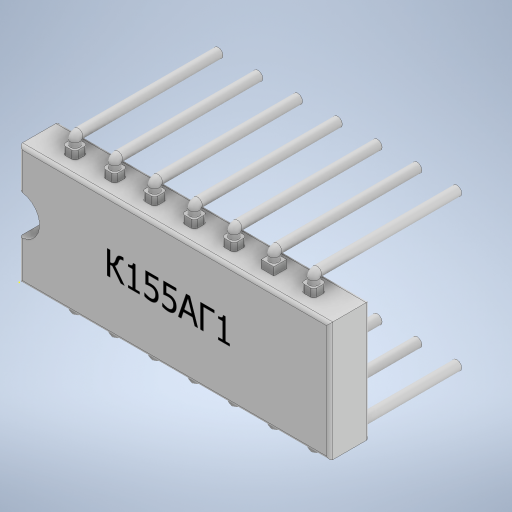
# Autodesk Inventor part: К155АГ1
Saved by Autodesk Inventor 2024 (Build 280153000, 153)
## iProperties
Created: 2023-12-19
Part Number: К155АГ1
Material: Generic
Document SubType Name: Sheet Metal
Designer: user
Density: 1 g/cm^3
Sheet Metal Rule: Default
Appearance: Default
Author: user
Autodesk Inventor part; units mm, degrees
sketch "Sketch1" plane through (0, 0, 0) normal (0, 0, 1) x (1, 0, 0)
  line L0 (0, 0) -> (495.3, 0)
  line L1 (495.3, 0) -> (495.3, 190.5)
  line L2 (495.3, 190.5) -> (0, 190.5)
  line L3 (0, 190.5) -> (0, 127)
  line L4 (0, 0) -> (0, 63.5)
  arc A0 (0, 63.5) -> (0, 127) centre (0.6755, 95.25) ccw
  line L5 (0, 190.5) -> (57.15, 190.5)
  line L6 (57.15, 190.5) -> (57.15, 203.2)
  line L7 (46.99, 203.2) -> (67.31, 203.2)
  line L8 (67.31, 203.2) -> (67.31, 190.5)
  line L9 (67.31, 190.5) -> (46.99, 190.5)
  line L10 (46.99, 190.5) -> (46.99, 203.2)
  line L11 (57.15, 203.2) -> (120.65, 203.2)
  line L12 (120.65, 203.2) -> (184.15, 203.2)
  line L13 (184.15, 203.2) -> (247.65, 203.2)
  line L14 (247.65, 203.2) -> (311.15, 203.2)
  line L15 (311.15, 203.2) -> (374.65, 203.2)
  line L16 (374.65, 203.2) -> (438.15, 203.2)
  line L17 (438.15, 203.2) -> (495.3, 203.2)
  line L18 (120.65, 203.2) -> (110.49, 203.2)
  line L19 (110.49, 203.2) -> (110.49, 190.5)
  line L20 (110.49, 190.5) -> (120.65, 190.5)
  line L21 (120.65, 190.5) -> (120.65, 203.2)
  line L22 (120.65, 203.2) -> (130.81, 203.2)
  line L23 (130.81, 203.2) -> (130.81, 190.5)
  line L24 (130.81, 190.5) -> (120.65, 190.5)
  line L25 (120.65, 190.5) -> (120.65, 203.2)
  line L26 (184.15, 203.2) -> (173.99, 203.2)
  line L27 (173.99, 203.2) -> (173.99, 190.5)
  line L28 (173.99, 190.5) -> (184.15, 190.5)
  line L29 (184.15, 190.5) -> (184.15, 203.2)
  line L30 (184.15, 203.2) -> (194.31, 203.2)
  line L31 (194.31, 203.2) -> (194.31, 190.5)
  line L32 (194.31, 190.5) -> (184.15, 190.5)
  line L33 (184.15, 190.5) -> (184.15, 203.2)
  line L34 (247.65, 203.2) -> (237.49, 203.2)
  line L35 (237.49, 203.2) -> (237.49, 190.5)
  line L36 (237.49, 190.5) -> (247.65, 190.5)
  line L37 (247.65, 190.5) -> (247.65, 203.2)
  line L38 (247.65, 203.2) -> (257.81, 203.2)
  line L39 (257.81, 203.2) -> (257.81, 190.5)
  line L40 (257.81, 190.5) -> (247.65, 190.5)
  line L41 (247.65, 190.5) -> (247.65, 203.2)
  line L42 (311.15, 203.2) -> (300.99, 203.2)
  line L43 (300.99, 203.2) -> (300.99, 190.5)
  line L44 (300.99, 190.5) -> (311.15, 190.5)
  line L45 (311.15, 190.5) -> (311.15, 203.2)
  line L46 (311.15, 203.2) -> (321.31, 203.2)
  line L47 (321.31, 203.2) -> (321.31, 190.5)
  line L48 (321.31, 190.5) -> (311.15, 190.5)
  line L49 (311.15, 190.5) -> (311.15, 203.2)
  line L50 (374.65, 203.2) -> (384.81, 203.2)
  line L51 (384.81, 203.2) -> (384.81, 190.5)
  line L52 (384.81, 190.5) -> (374.65, 190.5)
  line L53 (374.65, 190.5) -> (374.65, 203.2)
  line L54 (374.65, 203.2) -> (364.49, 203.2)
  line L55 (364.49, 203.2) -> (364.49, 190.5)
  line L56 (364.49, 190.5) -> (374.65, 190.5)
  line L57 (374.65, 190.5) -> (374.65, 203.2)
  line L58 (438.15, 203.2) -> (448.31, 203.2)
  line L59 (448.31, 203.2) -> (448.31, 190.5)
  line L60 (448.31, 190.5) -> (438.15, 190.5)
  line L61 (438.15, 190.5) -> (438.15, 203.2)
  line L62 (438.15, 203.2) -> (427.99, 203.2)
  line L63 (427.99, 203.2) -> (427.99, 190.5)
  line L64 (427.99, 190.5) -> (438.15, 190.5)
  line L65 (438.15, 190.5) -> (438.15, 203.2)
  line L66 (0, 0) -> (57.15, 0)
  line L67 (57.15, 0) -> (120.65, 0)
  line L68 (120.65, 0) -> (184.15, 0)
  line L69 (184.15, 0) -> (247.65, 0)
  line L70 (247.65, 0) -> (311.15, 0)
  line L71 (311.15, 0) -> (374.65, 0)
  line L72 (374.65, 0) -> (438.15, 0)
  line L73 (438.15, 0) -> (495.3, 0)
  line L74 (57.15, 0) -> (46.99, 0)
  line L75 (46.99, 0) -> (46.99, -12.7)
  line L76 (46.99, -12.7) -> (57.15, -12.7)
  line L77 (57.15, -12.7) -> (57.15, 0)
  line L78 (57.15, 0) -> (67.31, 0)
  line L79 (67.31, 0) -> (67.31, -12.7)
  line L80 (67.31, -12.7) -> (57.15, -12.7)
  line L81 (57.15, -12.7) -> (57.15, 0)
  line L82 (120.65, 0) -> (110.49, 0)
  line L83 (110.49, 0) -> (110.49, -12.7)
  line L84 (110.49, -12.7) -> (120.65, -12.7)
  line L85 (120.65, -12.7) -> (120.65, 0)
  line L86 (120.65, 0) -> (130.81, 0)
  line L87 (130.81, 0) -> (130.81, -12.7)
  line L88 (130.81, -12.7) -> (120.65, -12.7)
  line L89 (120.65, -12.7) -> (120.65, 0)
  line L90 (184.15, 0) -> (194.31, 0)
  line L91 (194.31, 0) -> (194.31, -12.7)
  line L92 (194.31, -12.7) -> (184.15, -12.7)
  line L93 (184.15, -12.7) -> (184.15, 0)
  line L94 (184.15, 0) -> (173.99, 0)
  line L95 (173.99, 0) -> (173.99, -12.7)
  line L96 (173.99, -12.7) -> (184.15, -12.7)
  line L97 (184.15, -12.7) -> (184.15, 0)
  line L98 (247.65, 0) -> (257.81, 0)
  line L99 (257.81, 0) -> (257.81, -12.7)
  line L100 (257.81, -12.7) -> (247.65, -12.7)
  line L101 (247.65, -12.7) -> (247.65, 0)
  line L102 (247.65, 0) -> (237.49, 0)
  line L103 (237.49, 0) -> (237.49, -12.7)
  line L104 (237.49, -12.7) -> (247.65, -12.7)
  line L105 (247.65, -12.7) -> (247.65, 0)
  line L106 (311.15, 0) -> (321.31, 0)
  line L107 (321.31, 0) -> (321.31, -12.7)
  line L108 (321.31, -12.7) -> (311.15, -12.7)
  line L109 (311.15, -12.7) -> (311.15, 0)
  line L110 (311.15, 0) -> (300.99, 0)
  line L111 (300.99, 0) -> (300.99, -12.7)
  line L112 (300.99, -12.7) -> (311.15, -12.7)
  line L113 (311.15, -12.7) -> (311.15, 0)
  line L114 (374.65, 0) -> (384.81, 0)
  line L115 (384.81, 0) -> (384.81, -12.7)
  line L116 (384.81, -12.7) -> (374.65, -12.7)
  line L117 (374.65, -12.7) -> (374.65, 0)
  line L118 (374.65, 0) -> (364.49, 0)
  line L119 (364.49, 0) -> (364.49, -12.7)
  line L120 (364.49, -12.7) -> (374.65, -12.7)
  line L121 (374.65, -12.7) -> (374.65, 0)
  line L122 (438.15, 0) -> (448.31, 0)
  line L123 (448.31, 0) -> (448.31, -12.7)
  line L124 (448.31, -12.7) -> (438.15, -12.7)
  line L125 (438.15, -12.7) -> (438.15, 0)
  line L126 (438.15, 0) -> (427.99, 0)
  line L127 (427.99, 0) -> (427.99, -12.7)
  line L128 (427.99, -12.7) -> (438.15, -12.7)
  line L129 (438.15, -12.7) -> (438.15, 0)
  dimension "d0" = 495.3
  dimension "d1" = 190.5
  dimension "d2" = 495.3
  dimension "d3" = 63.5
  dimension "d4" = 63.5
  dimension "d5" = 57.15
  dimension "d6" = 12.7
  dimension "d8" = 10.16
  dimension "d9" = 63.5
  dimension "d10" = 63.5
  dimension "d11" = 63.5
  dimension "d12" = 63.5
  dimension "d13" = 63.5
  dimension "d14" = 63.5
  dimension "d15" = 57.15
  dimension "d16" = 10.16
  dimension "d17" = 12.7
  dimension "d18" = 10.16
  dimension "d19" = 12.7
  dimension "d20" = 10.16
  dimension "d21" = 10.16
  dimension "d22" = 12.7
  dimension "d23" = 10.16
  dimension "d24" = 12.7
  dimension "d25" = 10.16
  dimension "d26" = 12.7
  dimension "d27" = 10.16
  dimension "d28" = 12.7
  dimension "d29" = 10.16
  dimension "d30" = 12.7
  dimension "d31" = 10.16
  dimension "d32" = 12.7
  dimension "d33" = 10.16
  dimension "d34" = 12.7
  dimension "d35" = 10.16
  dimension "d36" = 12.7
  dimension "d37" = 10.16
  dimension "d38" = 12.7
  dimension "d39" = 57.15
  dimension "d40" = 63.5
  dimension "d41" = 63.5
  dimension "d42" = 63.5
  dimension "d43" = 63.5
  dimension "d44" = 63.5
  dimension "d45" = 63.5
  dimension "d46" = 57.15
  dimension "d47" = 10.16
  dimension "d48" = 12.7
  dimension "d49" = 10.16
  dimension "d50" = 12.7
  dimension "d51" = 10.16
  dimension "d52" = 12.7
  dimension "d53" = 10.16
  dimension "d54" = 12.7
  dimension "d55" = 10.16
  dimension "d56" = 12.7
  dimension "d57" = 10.16
  dimension "d58" = 12.7
  dimension "d59" = 10.16
  dimension "d60" = 12.7
  dimension "d61" = 10.16
  dimension "d62" = 12.7
  dimension "d63" = 10.16
  dimension "d64" = 12.7
  constraints: 258 end point, 54 parallel, 30 perpendicular, 27 horizontal, 9 point on line, 3 vertical, 2 point on circle, 1 centre point, 1 collinear, 10 other
  measures "d0" distance of L4.start L1.start
  measures "d1" distance of L1.start L1.end
  measures "d2" distance of L1.end L2.end
  measures "d3" distance of L2.end L3.end
  measures "d4" distance of L4.start L4.end
  measures "d5" distance of L2.end L5.end
  measures "d6" distance of L5.end L6.end
  measures "d8" distance of L6.end L7.start
  measures "d9" distance of L6.end L11.end
  measures "d10" distance of L11.end L12.end
  measures "d11" distance of L12.end L13.end
  measures "d12" distance of L13.end L14.end
  measures "d13" distance of L14.end L15.end
  measures "d14" distance of L15.end L16.end
  measures "d15" distance of L16.end L17.end
  measures "d16" distance of L20.end L19.end
  measures "d17" distance of L19.end L18.end
  measures "d18" distance of L23.end L24.end
  measures "d19" distance of L22.end L23.end
  measures "d20" distance of L28.end L27.end
  measures "d21" distance of L31.end L32.end
  measures "d22" distance of L30.end L31.end
  measures "d23" distance of L36.end L35.end
  measures "d24" distance of L35.end L34.end
  measures "d25" distance of L39.end L40.end
  measures "d26" distance of L38.end L39.end
  measures "d27" distance of L44.end L43.end
  measures "d28" distance of L43.end L42.end
  measures "d29" distance of L47.end L48.end
  measures "d30" distance of L46.end L47.end
  measures "d31" distance of L51.end L52.end
  measures "d32" distance of L50.end L51.end
  measures "d33" distance of L56.end L55.end
  measures "d34" distance of L55.end L54.end
  measures "d35" distance of L59.end L60.end
  measures "d36" distance of L58.end L59.end
  measures "d37" distance of L64.end L63.end
  measures "d38" distance of L63.end L62.end
  measures "d39" distance of L4.start L66.end
  measures "d40" distance of L66.end L67.end
  measures "d41" distance of L67.end L68.end
  measures "d42" distance of L68.end L69.end
  measures "d43" distance of L69.end L70.end
  measures "d44" distance of L70.end L71.end
  measures "d45" distance of L71.end L72.end
  measures "d46" distance of L72.end L1.start
  measures "d47" distance of L76.end L75.end
  measures "d48" distance of L75.end L74.end
  measures "d49" distance of L79.end L80.end
  measures "d50" distance of L78.end L79.end
  measures "d51" distance of L84.end L83.end
  measures "d52" distance of L83.end L82.end
  measures "d53" distance of L87.end L88.end
  measures "d54" distance of L86.end L87.end
  measures "d55" distance of L91.end L92.end
  measures "d56" distance of L90.end L91.end
  measures "d57" distance of L96.end L95.end
  measures "d58" distance of L95.end L94.end
  measures "d59" distance of L99.end L100.end
  measures "d60" distance of L98.end L99.end
  measures "d61" distance of L104.end L103.end
  measures "d62" distance of L103.end L102.end
  measures "d63" distance of L107.end L108.end
  measures "d64" distance of L106.end L107.end
extrude "Extrusion1" add sketch "Sketch1" along normal mid plane 63.5 contours L4 A0 L3 L2 L1 L0
extrude "Extrusion2" add sketch "Sketch1" along normal mid plane 20.32 contours L0 L77 L76 L75 | L0 L79 L80 L77 | L0 L85 L84 L83 | L10 L7 L6 L2 | L0 L87 L88 L85 | L6 L7 L8 L2 | L0 L93 L96 L95 | L19 L11 L21 L2 | L0 L91 L92 L93 | L21 L12 L23 L2 | L0 L101 L104 L103 | L27 L12 L29 L2 | L0 L99 L100 L101 | L29 L13 L31 L2 | L0 L109 L112 L111 | L35 L13 L37 L2 | L0 L107 L108 L109 | L37 L14 L39 L2 | L0 L117 L120 L119 | L43 L14 L45 L2 | L0 L115 L116 L117 | L45 L15 L47 L2 | L0 L125 L128 L127 | L55 L15 L53 L2 | L0 L123 L124 L125 | L53 L16 L51 L2 | L63 L16 L61 L2 | L61 L17 L59 L2
fillet "Fillet1" radius 5.08 62 edges at (67.31, 196.85, 10.16) (67.31, 196.85, -10.16) (46.99, 196.85, -10.16) (46.99, 196.85, 10.16) (110.49, 196.85, 10.16) (130.81, 196.85, 10.16) (110.49, 196.85, -10.16) (130.81, 196.85, -10.16) (173.99, 196.85, 10.16) (173.99, 196.85, -10.16) (194.31, 196.85, -10.16) (194.31, 196.85, 10.16) (237.49, 196.85, 10.16) (257.81, 196.85, 10.16) (237.49, 196.85, -10.16) (257.81, 196.85, -10.16) (300.99, 196.85, 10.16) (321.31, 196.85, 10.16) (300.99, 196.85, -10.16) (321.31, 196.85, -10.16) (427.99, 196.85, 10.16) (448.31, 196.85, 10.16) (448.31, 196.85, -10.16) (427.99, 196.85, -10.16) (46.99, -6.35, 10.16) (46.99, -6.35, -10.16) (67.31, -6.35, -10.16) (67.31, -6.35, 10.16) (110.49, -6.35, 10.16) (110.49, -6.35, -10.16) (130.81, -6.35, 10.16) (130.81, -6.35, -10.16) (173.99, -6.35, -10.16) (173.99, -6.35, 10.16) (194.31, -6.35, 10.16) (194.31, -6.35, -10.16) (237.49, -6.35, 10.16) (237.49, -6.35, -10.16) (257.81, -6.35, 10.16) (257.81, -6.35, -10.16) (300.99, -6.35, 10.16) (321.31, -6.35, 10.16) (300.99, -6.35, -10.16) (321.31, -6.35, -10.16) (364.49, -6.35, -10.16) (384.81, -6.35, -10.16) (364.49, -6.35, 10.16) (384.81, -6.35, 10.16) (427.99, -6.35, 10.16) (427.99, -6.35, -10.16) (448.31, -6.35, 10.16) (448.31, -6.35, -10.16) (247.65, 0, 31.75) (495.3, 95.25, 31.75) (247.65, 190.5, 31.75) (0, 31.75, 31.75) (0, 158.75, 31.75) (247.65, 0, -31.75) (0, 31.75, -31.75) (0, 158.75, -31.75) (495.3, 95.25, -31.75) (247.65, 190.5, -31.75)
ref_plane "Work Plane1" through (433.07, 203.2, 10.16) normal (0, 1, 0) x (1, 0, 0)
ref_plane "Work Plane2" through (364.49, 203.2, 10.16) normal (0, 1, 0) x (1, 0, 0)
ref_plane "Work Plane3" through (306.07, 203.2, -10.16) normal (0, 1, 0) x (1, 0, 0)
ref_plane "Work Plane4" through (242.57, 203.2, -10.16) normal (0, 1, 0) x (1, 0, 0)
ref_plane "Work Plane5" through (179.07, 203.2, -10.16) normal (0, 1, 0) x (1, 0, 0)
ref_plane "Work Plane6" through (115.57, 203.2, -10.16) normal (0, 1, 0) x (1, 0, 0)
ref_plane "Work Plane7" through (52.07, 203.2, 10.16) normal (0, 1, 0) x (1, 0, 0)
sketch "Sketch2" plane through (52.07, 203.2, 10.16) normal (0, 1, 0) x (1, 0, 0)
  line L0 (15.24, 5.08) -> (15.24, 15.24) projected
  circle A0 centre (5.08, 10.16) radius 7.62
  point P0 (-52.07, 10.16)
  dimension "d88" = 15.24
  constraints: 1 centre point
  measures "d88" diameter of A0
sketch "Sketch4" plane through (115.57, 203.2, -10.16) normal (0, 1, 0) x (1, 0, 0)
  line L0 (-5.08, -15.24) -> (-5.08, -5.08) projected
  circle A0 centre (5.08, -10.16) radius 7.62
  point P0 (-115.57, -10.16)
  dimension "d90" = 15.24
  constraints: 1 centre point
  measures "d90" diameter of A0
sketch "Sketch5" plane through (179.07, 203.2, -10.16) normal (0, 1, 0) x (1, 0, 0)
  circle A0 centre (5.08, -10.16) radius 7.62
  point P0 (-115.57, -10.16)
  dimension "d91" = 15.24
  constraints: 1 centre point
  measures "d91" diameter of A0
sketch "Sketch6" plane through (242.57, 203.2, -10.16) normal (0, 1, 0) x (1, 0, 0)
  circle A0 centre (5.08, -10.16) radius 7.62
  point P0 (-115.57, -10.16)
  dimension "d92" = 15.24
  constraints: 1 centre point
  measures "d92" diameter of A0
sketch "Sketch7" plane through (306.07, 203.2, -10.16) normal (0, 1, 0) x (1, 0, 0)
  circle A0 centre (5.08, -10.16) radius 7.62
  point P0 (-115.57, -10.16)
  dimension "d93" = 15.24
  constraints: 1 centre point
  measures "d93" diameter of A0
sketch "Sketch8" plane through (364.49, 203.2, 10.16) normal (0, 1, 0) x (1, 0, 0)
  circle A0 centre (10.133, 10.16) radius 7.62
  point P0 (-52.07, 10.16)
  dimension "d94" = 15.24
  constraints: 1 centre point
  measures "d94" diameter of A0
sketch "Sketch9" plane through (433.07, 203.2, 10.16) normal (0, 1, 0) x (1, 0, 0)
  circle A0 centre (5.08, 10.16) radius 7.62
  point P0 (-52.07, 10.16)
  dimension "d95" = 15.24
  constraints: 1 centre point
  measures "d95" diameter of A0
ref_plane "Work Plane8" through (438.15, 190.5, -5.08) normal (-1, 0, 0) x (0, 0, 1)
ref_plane "Work Plane9" through (374.65, 190.5, 10.16) normal (-1, 0, 0) x (0, 0, 1)
ref_plane "Work Plane10" through (311.15, 190.5, -5.08) normal (1, 0, 0) x (0, 0, -1)
ref_plane "Work Plane11" through (247.65, 190.5, -5.08) normal (1, 0, 0) x (0, 0, -1)
ref_plane "Work Plane12" through (184.15, 190.5, 5.08) normal (1, 0, 0) x (0, 0, -1)
ref_plane "Work Plane13" through (120.65, 190.5, -5.08) normal (1, 0, 0) x (0, 0, -1)
ref_plane "Work Plane14" through (57.15, 190.5, -5.08) normal (1, 0, 0) x (0, 0, -1)
sketch "Sketch10" plane through (184.15, 190.5, 5.08) normal (1, 0, 0) x (0, 0, -1)
  line L0 (0, 0) -> (10.16, 0) projected
  line L1 (5.08, 0) -> (5.08, 20.32)
  line L2 (10.16, 25.4) -> (233.68, 25.4)
  line L3 (5.08, 0) -> (5.08, -190.5)
  line L4 (5.08, -190.5) -> (5.08, -210.82)
  line L5 (10.16, -215.9) -> (233.68, -215.9)
  arc A0 (10.16, 25.4) -> (5.08, 20.32) centre (10.16, 20.32) ccw
  arc A1 (5.08, -210.82) -> (10.16, -215.9) centre (10.16, -210.82) ccw
  point P0 (5.08, 25.4)
  point P1 (5.08, -215.9)
  dimension "d97" = 25.4
  dimension "d98" = 228.6
  dimension "d99" = 25.4
  dimension "d100" = 228.6
  dimension "d101" = 5.08
  constraints: 10 end point, 5 point on line, 4 point on circle, 4 tangent, 2 centre point, 2 perpendicular, 2 vertical, 1 equal radius, 1 midpoint
  measures "d97" distance of L1.start point (5.08, 25.4)
  measures "d98" distance of point (5.08, 25.4) L2.end
  measures "d99" distance of L3.end point (5.08, -215.9)
  measures "d100" distance of point (5.08, -215.9) L5.end
  measures "d101" radius of A0
sketch "Sketch15" plane through (374.65, 190.5, 10.16) normal (-1, 0, 0) x (0, 0, 1)
  line L0 (-20.32, 0) -> (0, 0) projected
  line L1 (-10.16, 0) -> (-10.16, 20.32)
  line L2 (-15.24, 25.4) -> (-238.76, 25.4)
  line L3 (-10.16, 0) -> (-10.16, -190.5)
  line L4 (-10.16, -190.5) -> (-10.16, -210.82)
  line L5 (-15.24, -215.9) -> (-238.76, -215.9)
  arc A0 (-15.24, -215.9) -> (-10.16, -210.82) centre (-15.24, -210.82) ccw
  arc A1 (-10.16, 20.32) -> (-15.24, 25.4) centre (-15.24, 20.32) ccw
  point P0 (-10.16, 25.4)
  point P1 (-10.16, -215.9)
  dimension "d123" = 228.6
  dimension "d124" = 25.4
  dimension "d125" = 228.6
  dimension "d126" = 5.08
  constraints: 10 end point, 5 point on line, 4 point on circle, 4 tangent, 2 centre point, 2 perpendicular, 2 vertical, 1 equal radius, 1 midpoint
  measures "d123" distance of point (-10.16, 25.4) L2.end
  measures "d124" distance of L3.end point (-10.16, -215.9)
  measures "d125" distance of point (-10.16, -215.9) L5.end
  measures "d126" radius of A0
sketch "Sketch16" plane through (438.15, 190.5, -5.08) normal (-1, 0, 0) x (0, 0, 1)
  line L0 (5.0936, -0.0098) -> (5.0936, 20.32)
  line L1 (0.0136, 25.4) -> (-223.5064, 25.4)
  line L2 (5.0936, -0.0098) -> (5.0936, -190.5)
  line L3 (5.0936, -190.5) -> (5.0936, -210.82)
  line L4 (0.0136, -215.9) -> (-223.5064, -215.9)
  arc A0 (0.0136, -215.9) -> (5.0936, -210.82) centre (0.0136, -210.82) ccw
  arc A1 (5.0936, 20.32) -> (0.0136, 25.4) centre (0.0136, 20.32) ccw
  point P0 (5.0936, 25.4)
  point P1 (5.0936, -215.9)
  dimension "d127" = 228.6
  dimension "d128" = 25.4
  dimension "d129" = 228.6
  dimension "d130" = 5.08
  constraints: 10 end point, 5 point on line, 4 point on circle, 4 tangent, 2 centre point, 2 perpendicular, 2 vertical, 1 equal radius
  measures "d127" distance of point (5.094, 25.4) L1.end
  measures "d128" distance of L2.end point (5.094, -215.9)
  measures "d129" distance of point (5.094, -215.9) L4.end
  measures "d130" radius of A0
sweep "Sweep1" add profiles "Sketch9" path "Sketch16"
sweep "Sweep2" add profiles "Sketch8" path "Sketch15" path curves L2 A1 L1 L3 L4 A0 L5
sweep "Sweep3" add profiles "Sketch5" path "Sketch10" path curves L2 A0 L1 L3 L4 A1 L5
sketch "Sketch17" plane through (311.15, 190.5, -5.08) normal (1, 0, 0) x (0, 0, -1)
  line L0 (5.08, 0) -> (-15.24, 0) projected
  line L1 (-5.08, 0) -> (-5.08, 20.32)
  line L2 (0, 25.4) -> (223.52, 25.4)
  line L3 (-5.08, 0) -> (-5.08, -190.5)
  line L4 (-5.08, -190.5) -> (-5.08, -210.82)
  line L5 (0, -215.9) -> (223.52, -215.9)
  arc A0 (0, 25.4) -> (-5.08, 20.32) centre (0, 20.32) ccw
  arc A1 (-5.08, -210.82) -> (0, -215.9) centre (0, -210.82) ccw
  point P0 (-5.08, 25.4)
  point P1 (-5.08, -215.9)
  dimension "d137" = 25.4
  dimension "d138" = 228.6
  dimension "d139" = 25.4
  dimension "d140" = 228.6
  dimension "d141" = 5.08
  constraints: 10 end point, 5 point on line, 4 point on circle, 4 tangent, 2 centre point, 2 perpendicular, 2 vertical, 1 equal radius, 1 midpoint
  measures "d137" distance of L1.start point (-5.08, 25.4)
  measures "d138" distance of point (-5.08, 25.4) L2.end
  measures "d139" distance of L3.end point (-5.08, -215.9)
  measures "d140" distance of point (-5.08, -215.9) L5.end
  measures "d141" radius of A0
sweep "Sweep4" add profiles "Sketch7" path "Sketch17" path curves L2 A0 L1 L3 L4 A1 L5
sketch "Sketch18" plane through (247.65, 190.5, -5.08) normal (1, 0, 0) x (0, 0, -1)
  line L0 (-5.08, 0) -> (-5.08, 20.32)
  line L1 (0, 25.4) -> (223.52, 25.4)
  line L2 (-5.08, 0) -> (-5.08, -190.5)
  line L3 (-5.08, -190.5) -> (-5.08, -210.82)
  line L4 (0, -215.9) -> (223.52, -215.9)
  arc A0 (0, 25.4) -> (-5.08, 20.32) centre (0, 20.32) ccw
  arc A1 (-5.08, -210.82) -> (0, -215.9) centre (0, -210.82) ccw
  point P0 (-5.08, 25.4)
  point P1 (-5.08, -215.9)
  dimension "d144" = 25.4
  dimension "d145" = 228.6
  dimension "d146" = 25.4
  dimension "d147" = 228.6
  dimension "d148" = 5.08
  constraints: 10 end point, 5 point on line, 4 point on circle, 4 tangent, 2 centre point, 2 perpendicular, 2 vertical, 1 equal radius
  measures "d144" distance of L0.start point (-5.08, 25.4)
  measures "d145" distance of point (-5.08, 25.4) L1.end
  measures "d146" distance of L2.end point (-5.08, -215.9)
  measures "d147" distance of point (-5.08, -215.9) L4.end
  measures "d148" radius of A0
sketch "Sketch19" plane through (120.65, 190.5, -5.08) normal (1, 0, 0) x (0, 0, -1)
  line L0 (-5.08, 0) -> (-5.08, 20.32)
  line L1 (0, 25.4) -> (223.52, 25.4)
  line L2 (-5.08, 0) -> (-5.08, -190.5)
  line L3 (-5.08, -190.5) -> (-5.08, -210.82)
  line L4 (0, -215.9) -> (223.52, -215.9)
  arc A0 (0, 25.4) -> (-5.08, 20.32) centre (0, 20.32) ccw
  arc A1 (-5.08, -210.82) -> (0, -215.9) centre (0, -210.82) ccw
  point P0 (-5.08, 25.4)
  point P1 (-5.08, -215.9)
  dimension "d149" = 25.4
  dimension "d150" = 228.6
  dimension "d151" = 25.4
  dimension "d152" = 228.6
  dimension "d153" = 5.08
  constraints: 10 end point, 5 point on line, 4 point on circle, 4 tangent, 2 centre point, 2 perpendicular, 2 vertical, 1 equal radius
  measures "d149" distance of L0.start point (-5.08, 25.4)
  measures "d150" distance of point (-5.08, 25.4) L1.end
  measures "d151" distance of L2.end point (-5.08, -215.9)
  measures "d152" distance of point (-5.08, -215.9) L4.end
  measures "d153" radius of A0
sketch "Sketch20" plane through (57.15, 190.5, -5.08) normal (1, 0, 0) x (0, 0, -1)
  line L0 (-5.08, 0) -> (-5.08, 20.32)
  line L1 (0, 25.4) -> (223.52, 25.4)
  line L2 (-5.08, 0) -> (-5.08, -190.5)
  line L3 (-5.08, -190.5) -> (-5.08, -210.82)
  line L4 (0, -215.9) -> (223.52, -215.9)
  arc A0 (0, 25.4) -> (-5.08, 20.32) centre (0, 20.32) ccw
  arc A1 (-5.08, -210.82) -> (0, -215.9) centre (0, -210.82) ccw
  point P0 (-5.08, 25.4)
  point P1 (-5.08, -215.9)
  dimension "d154" = 25.4
  dimension "d155" = 228.6
  dimension "d156" = 25.4
  dimension "d157" = 228.6
  dimension "d158" = 5.08
  constraints: 10 end point, 5 point on line, 4 point on circle, 4 tangent, 2 centre point, 2 perpendicular, 2 vertical, 1 equal radius
  measures "d154" distance of L0.start point (-5.08, 25.4)
  measures "d155" distance of point (-5.08, 25.4) L1.end
  measures "d156" distance of L2.end point (-5.08, -215.9)
  measures "d157" distance of point (-5.08, -215.9) L4.end
  measures "d158" radius of A0
sweep "Sweep5" add profiles "Sketch6" path "Sketch18"
sweep "Sweep6" add profiles "Sketch4" path "Sketch19"
sweep "Sweep7" add profiles "Sketch2" path "Sketch20"
sketch "Sketch21" plane through (0, 0, 31.75) normal (0, 0, 1) x (1, 0, 0)
  line L0 (136.2776, 117.6449) -> (415.6011, 117.6449) construction
  line L1 (415.6011, 117.6449) -> (415.6011, 52.0579) construction
  line L2 (415.6011, 52.0579) -> (136.2776, 52.0579) construction
  line L3 (136.2776, 52.0579) -> (136.2776, 117.6449) construction
  point P0 (0, 0)
  constraints: 2 other
equation "\"BendRadius\" = Thickness"
equation "\"BendReliefWidth\" = Thickness"
equation "\"BendReliefDepth\" = 0.5 * Thickness"
equation "\"CornerReliefSize\" = 4 * Thickness"
equation "\"MinimumRemnant\" = 2 * Thickness"
equation "\"TransitionRadius\" = BendRadius"
equation "\"JacobiRadiusSize\" = BendRadius"
equation "\"GapSize\" = Thickness"
equation "\"Thickness\" = 3.048"
body "Solid1"
